Autodesk Fusion 360 part; units mm, degrees
(part 2 of 2)
  spline S357 degree 3 poles (-3.8049, -47.8973) (-3.3486, -49.266) (-3.3114, -49.4383) (-3.4138, -49.7828) knots 0 0 0 0 1 1 1 1
  spline S358 degree 3 poles (-3.4138, -49.7828) (-3.5255, -50.1506) (-3.4464, -50.4812) (-3.2508, -50.4812) knots 0 0 0 0 1 1 1 1
  spline S359 degree 3 poles (-3.2508, -50.4812) (-3.1484, -50.4812) (-3.1065, -50.416) (-3.0693, -50.2018) knots 0 0 0 0 1 1 1 1
  spline S360 degree 3 poles (-3.0693, -50.2018) (-3.032, -50.0249) (-3.0367, -50.0203) (-2.883, -50.5045) knots 0 0 0 0 1 1 1 1
  spline S361 degree 3 poles (-2.883, -50.5045) (-2.8225, -50.6814) (-2.7294, -50.9235) (-2.6689, -51.0399) knots 0 0 0 0 1 1 1 1
  spline S362 degree 3 poles (-2.6689, -51.0399) (-2.5385, -51.282) (-2.5292, -51.403) (-2.6316, -51.4449) knots 0 0 0 0 1 1 1 1
  spline S363 degree 3 poles (-2.6316, -51.4449) (-2.6735, -51.4589) (-2.9482, -51.4403) (-3.2415, -51.3984) knots 0 0 0 0 1 1 1 1
  spline S364 degree 3 poles (-3.2415, -51.3984) (-3.7863, -51.3192) (-4.303, -51.1237) (-4.4334, -50.9514) knots 0 0 0 0 1 1 1 1
  spline S365 degree 3 poles (-4.4334, -50.9514) (-4.466, -50.9095) (-4.587, -50.7978) (-4.7034, -50.7) knots 0 0 0 0 1 1 1 1
  spline S366 degree 3 poles (-4.7034, -50.7) (-4.9641, -50.4905) (-5.2156, -50.0249) (-5.2481, -49.6897) knots 0 0 0 0 1 1 1 1
  spline S367 degree 3 poles (-5.2481, -49.6897) (-5.29, -49.2474) (-4.9921, -48.158) (-4.7314, -47.8274) knots 0 0 0 0 1 1 1 1
  spline S368 degree 3 poles (-4.7314, -47.8274) (-4.466, -47.4783) (-4.1634, -47.1756) (-4.1028, -47.185) knots 0 0 0 0 1 1 1 1
  spline S369 degree 3 poles (-4.1028, -47.185) (-4.0656, -47.1943) (-3.9399, -47.5015) (-3.8049, -47.8973) knots 0 0 0 0 1 1 1 1
  spline S370 degree 3 poles (6.2235, -48.8005) (6.1909, -48.847) (5.9395, -48.9914) (5.2179, -49.3731) knots 0 0 0 0 1 1 1 1
  spline S371 degree 3 poles (5.2179, -49.3731) (4.9758, -49.5035) (4.7197, -49.6478) (4.6545, -49.6944) knots 0 0 0 0 1 1 1 1
  spline S372 degree 3 poles (4.6545, -49.6944) (4.5847, -49.7409) (4.5149, -49.7828) (4.5009, -49.7828) knots 0 0 0 0 1 1 1 1
  spline S373 degree 3 poles (4.5009, -49.7828) (4.4683, -49.7828) (4.026, -50.0482) (3.5185, -50.3695) knots 0 0 0 0 1 1 1 1
  spline S374 degree 3 poles (3.5185, -50.3695) (3.3416, -50.4812) (3.0902, -50.6348) (2.9645, -50.7047) knots 0 0 0 0 1 1 1 1
  spline S375 degree 3 poles (2.9645, -50.7047) (2.8388, -50.7745) (2.6619, -50.8955) (2.5688, -50.97) knots 0 0 0 0 1 1 1 1
  spline S376 degree 3 poles (2.5688, -50.97) (2.4757, -51.0492) (2.2569, -51.2028) (2.0753, -51.3146) knots 0 0 0 0 1 1 1 1
  spline S377 degree 3 poles (2.0753, -51.3146) (1.8984, -51.4263) (1.6982, -51.5567) (1.633, -51.6032) knots 0 0 0 0 1 1 1 1
  spline S378 degree 3 poles (1.633, -51.6032) (1.5678, -51.6498) (1.3909, -51.7662) (1.2373, -51.8639) knots 0 0 0 0 1 1 1 1
  spline S379 degree 3 poles (1.2373, -51.8639) (1.0836, -51.957) (0.916, -52.0781) (0.8648, -52.1247) knots 0 0 0 0 1 1 1 1
  spline S380 degree 3 poles (0.8648, -52.1247) (0.8136, -52.1712) (0.7158, -52.241) (0.6506, -52.2829) knots 0 0 0 0 1 1 1 1
  spline S381 degree 3 poles (0.6506, -52.2829) (0.3573, -52.4599) (0.3853, -52.6973) (0.6925, -52.6414) knots 0 0 0 0 1 1 1 1
  spline S382 degree 3 poles (0.6925, -52.6414) (0.8089, -52.6182) (0.8695, -52.6275) (0.9067, -52.674) knots 0 0 0 0 1 1 1 1
  spline S383 degree 3 poles (0.9067, -52.674) (1.0138, -52.809) (1.4468, -53.1396) (1.6051, -53.2048) knots 0 0 0 0 1 1 1 1
  spline S384 degree 3 poles (1.6051, -53.2048) (2.0054, -53.3724) (2.7224, -53.5074) (3.2206, -53.5074) knots 0 0 0 0 1 1 1 1
  spline S385 degree 3 poles (3.2206, -53.5074) (3.6955, -53.5074) (3.7187, -53.5027) (4.0819, -53.3258) knots 0 0 0 0 1 1 1 1
  spline S386 degree 3 poles (4.0819, -53.3258) (4.445, -53.1489) (4.6359, -53.0046) (4.9897, -52.6554) knots 0 0 0 0 1 1 1 1
  spline S387 degree 3 poles (4.9897, -52.6554) (5.162, -52.4878) (5.4972, -51.9803) (5.4972, -51.8919) knots 0 0 0 0 1 1 1 1
  spline S388 degree 3 poles (5.4972, -51.8919) (5.4972, -51.8686) (5.5577, -51.7243) (5.6322, -51.5706) knots 0 0 0 0 1 1 1 1
  spline S389 degree 3 poles (5.6322, -51.5706) (5.8138, -51.1935) (5.9255, -50.4626) (5.8836, -49.8666) knots 0 0 0 0 1 1 1 1
  line L38 (5.8836, -49.8666) -> (5.8557, -49.4243)
  line L39 (5.8557, -49.4243) -> (6.0187, -49.3033)
  spline S390 degree 3 poles (6.0187, -49.3033) (6.1071, -49.2335) (6.2002, -49.1776) (6.2282, -49.1776) knots 0 0 0 0 1 1 1 1
  spline S391 degree 3 poles (6.2282, -49.1776) (6.2514, -49.1776) (6.3213, -49.1264) (6.3818, -49.0612) knots 0 0 0 0 1 1 1 1
  spline S392 degree 3 poles (6.3818, -49.0612) (6.4703, -48.9634) (6.4842, -48.9215) (6.447, -48.861) knots 0 0 0 0 1 1 1 1
  spline S393 degree 3 poles (6.447, -48.861) (6.3865, -48.7679) (6.2608, -48.7353) (6.2235, -48.8005) knots 0 0 0 0 1 1 1 1
  spline S394 degree 3 poles (5.5298, -49.7177) (5.5438, -49.7596) (5.5345, -50.0668) (5.5019, -50.4067) knots 0 0 0 0 1 1 1 1
  spline S395 degree 3 poles (5.5019, -50.4067) (5.4507, -51.0352) (5.3203, -51.4915) (5.0596, -52.0036) knots 0 0 0 0 1 1 1 1
  spline S396 degree 3 poles (5.0596, -52.0036) (4.892, -52.3342) (4.4404, -52.7299) (3.9608, -52.972) knots 0 0 0 0 1 1 1 1
  spline S397 degree 3 poles (3.9608, -52.972) (3.742, -53.0837) (3.6303, -53.107) (3.2113, -53.1256) knots 0 0 0 0 1 1 1 1
  spline S398 degree 3 poles (3.2113, -53.1256) (2.8062, -53.1396) (2.6572, -53.1256) (2.3593, -53.0418) knots 0 0 0 0 1 1 1 1
  spline S399 degree 3 poles (2.3593, -53.0418) (1.7633, -52.8742) (1.1674, -52.5483) (1.1674, -52.3854) knots 0 0 0 0 1 1 1 1
  spline S400 degree 3 poles (1.1674, -52.3854) (1.1674, -52.3621) (1.2326, -52.3155) (1.3071, -52.2923) knots 0 0 0 0 1 1 1 1
  spline S401 degree 3 poles (1.3071, -52.2923) (1.3862, -52.2643) (1.4468, -52.2224) (1.4468, -52.1991) knots 0 0 0 0 1 1 1 1
  spline S402 degree 3 poles (1.4468, -52.1991) (1.4468, -52.1759) (1.5026, -52.1293) (1.5771, -52.1014) knots 0 0 0 0 1 1 1 1
  spline S403 degree 3 poles (1.5771, -52.1014) (1.647, -52.0688) (1.7633, -51.9943) (1.8332, -51.9384) knots 0 0 0 0 1 1 1 1
  spline S404 degree 3 poles (1.8332, -51.9384) (1.9077, -51.8779) (1.9868, -51.8313) (2.0101, -51.8313) knots 0 0 0 0 1 1 1 1
  spline S405 degree 3 poles (2.0101, -51.8313) (2.038, -51.8313) (2.1032, -51.7755) (2.1591, -51.7103) knots 0 0 0 0 1 1 1 1
  line L40 (2.1591, -51.7103) -> (2.2615, -51.5939)
  line L41 (2.2615, -51.5939) -> (2.2615, -51.8313)
  spline S406 degree 3 poles (2.2615, -51.8313) (2.2615, -52.0874) (2.3174, -52.1572) (2.4943, -52.12) knots 0 0 0 0 1 1 1 1
  spline S407 degree 3 poles (2.4943, -52.12) (2.62, -52.0967) (2.7131, -51.8919) (2.7829, -51.4822) knots 0 0 0 0 1 1 1 1
  spline S408 degree 3 poles (2.7829, -51.4822) (2.8202, -51.2401) (2.8295, -51.2308) (3.3137, -50.9468) knots 0 0 0 0 1 1 1 1
  spline S409 degree 3 poles (3.3137, -50.9468) (3.4254, -50.8816) (3.6908, -50.714) (3.9096, -50.5696) knots 0 0 0 0 1 1 1 1
  spline S410 degree 3 poles (3.9096, -50.5696) (4.1331, -50.4253) (4.4357, -50.2391) (4.5894, -50.1553) knots 0 0 0 0 1 1 1 1
  spline S411 degree 3 poles (4.5894, -50.1553) (4.743, -50.0715) (4.9059, -49.9737) (4.9525, -49.9318) knots 0 0 0 0 1 1 1 1
  spline S412 degree 3 poles (4.9525, -49.9318) (5.0736, -49.8247) (5.3669, -49.6525) (5.4414, -49.6478) knots 0 0 0 0 1 1 1 1
  spline S413 degree 3 poles (5.4414, -49.6478) (5.4739, -49.6432) (5.5112, -49.6758) (5.5298, -49.7177) knots 0 0 0 0 1 1 1 1
  spline S414 degree 3 poles (-7.2268, -49.6013) (-7.3246, -49.6571) (-7.3246, -49.7689) (-7.2315, -50.0948) knots 0 0 0 0 1 1 1 1
  spline S415 degree 3 poles (-7.2315, -50.0948) (-7.1616, -50.3369) (-7.1616, -50.3648) (-7.2548, -50.7093) knots 0 0 0 0 1 1 1 1
  spline S416 degree 3 poles (-7.2548, -50.7093) (-7.4084, -51.2773) (-7.3805, -52.3714) (-7.1896, -53.2048) knots 0 0 0 0 1 1 1 1
  spline S417 degree 3 poles (-7.1896, -53.2048) (-7.1384, -53.4189) (-6.9521, -53.8845) (-6.7659, -54.2523) knots 0 0 0 0 1 1 1 1
  spline S418 degree 3 poles (-6.7659, -54.2523) (-6.4074, -54.96) (-4.9409, -56.3613) (-4.2285, -56.6826) knots 0 0 0 0 1 1 1 1
  spline S419 degree 3 poles (-4.2285, -56.6826) (-4.1308, -56.7245) (-3.9958, -56.8036) (-3.9213, -56.8548) knots 0 0 0 0 1 1 1 1
  spline S420 degree 3 poles (-3.9213, -56.8548) (-3.7769, -56.9619) (-3.0739, -57.2459) (-2.3476, -57.4834) knots 0 0 0 0 1 1 1 1
  spline S421 degree 3 poles (-2.3476, -57.4834) (-1.5282, -57.7581) (-0.5878, -57.8977) (0.3992, -57.8931) knots 0 0 0 0 1 1 1 1
  spline S422 degree 3 poles (0.3992, -57.8931) (1.0091, -57.8931) (1.1721, -57.8744) (1.6702, -57.7534) knots 0 0 0 0 1 1 1 1
  spline S423 degree 3 poles (1.6702, -57.7534) (2.0753, -57.6556) (2.3174, -57.5672) (2.5083, -57.4554) knots 0 0 0 0 1 1 1 1
  spline S424 degree 3 poles (2.5083, -57.4554) (2.6526, -57.3623) (2.89, -57.232) (3.0297, -57.1621) knots 0 0 0 0 1 1 1 1
  spline S425 degree 3 poles (3.0297, -57.1621) (3.2951, -57.0271) (3.7001, -56.7291) (4.0074, -56.4405) knots 0 0 0 0 1 1 1 1
  spline S426 degree 3 poles (4.0074, -56.4405) (4.3147, -56.1518) (5.1713, -54.9739) (5.1713, -54.8389) knots 0 0 0 0 1 1 1 1
  spline S427 degree 3 poles (5.1713, -54.8389) (5.1713, -54.6853) (5.3063, -54.4944) (5.6881, -54.1033) knots 0 0 0 0 1 1 1 1
  spline S428 degree 3 poles (5.6881, -54.1033) (6.1164, -53.6703) (6.1956, -53.5353) (6.0559, -53.4608) knots 0 0 0 0 1 1 1 1
  spline S429 degree 3 poles (6.0559, -53.4608) (5.9907, -53.4236) (5.9162, -53.4655) (5.6788, -53.6797) knots 0 0 0 0 1 1 1 1
  spline S430 degree 3 poles (5.6788, -53.6797) (5.5158, -53.824) (5.3715, -53.9543) (5.3575, -53.973) knots 0 0 0 0 1 1 1 1
  spline S431 degree 3 poles (5.3575, -53.973) (5.2598, -54.1126) (4.054, -54.5596) (3.472, -54.676) knots 0 0 0 0 1 1 1 1
  spline S432 degree 3 poles (3.472, -54.676) (2.8062, -54.8063) (2.4012, -54.825) (1.6097, -54.7691) knots 0 0 0 0 1 1 1 1
  spline S433 degree 3 poles (1.6097, -54.7691) (0.4877, -54.6853) (-0.1781, -54.5922) (-0.6018, -54.4572) knots 0 0 0 0 1 1 1 1
  spline S434 degree 3 poles (-0.6018, -54.4572) (-0.8206, -54.392) (-1.1837, -54.2849) (-1.4118, -54.2244) knots 0 0 0 0 1 1 1 1
  spline S435 degree 3 poles (-1.4118, -54.2244) (-2.3989, -53.973) (-3.8747, -53.3398) (-4.3961, -52.9487) knots 0 0 0 0 1 1 1 1
  spline S436 degree 3 poles (-4.3961, -52.9487) (-4.5219, -52.8509) (-4.7127, -52.7252) (-4.8152, -52.6694) knots 0 0 0 0 1 1 1 1
  spline S437 degree 3 poles (-4.8152, -52.6694) (-5.0759, -52.525) (-5.2295, -52.3854) (-5.602, -51.9757) knots 0 0 0 0 1 1 1 1
  spline S438 degree 3 poles (-5.602, -51.9757) (-5.7789, -51.7801) (-6.0024, -51.5334) (-6.1001, -51.4263) knots 0 0 0 0 1 1 1 1
  spline S439 degree 3 poles (-6.1001, -51.4263) (-6.2026, -51.3192) (-6.2817, -51.2168) (-6.2817, -51.2028) knots 0 0 0 0 1 1 1 1
  spline S440 degree 3 poles (-6.2817, -51.2028) (-6.2817, -51.1842) (-6.3562, -51.0585) (-6.4493, -50.9188) knots 0 0 0 0 1 1 1 1
  spline S441 degree 3 poles (-6.4493, -50.9188) (-6.6542, -50.6115) (-6.9056, -50.1041) (-6.9847, -49.8387) knots 0 0 0 0 1 1 1 1
  spline S442 degree 3 poles (-6.9847, -49.8387) (-7.0546, -49.6013) (-7.1151, -49.5407) (-7.2268, -49.6013) knots 0 0 0 0 1 1 1 1
  spline S443 degree 3 poles (-6.7659, -51.2028) (-6.6681, -51.403) (-5.9791, -52.2085) (-5.8161, -52.3109) knots 0 0 0 0 1 1 1 1
  spline S444 degree 3 poles (-5.8161, -52.3109) (-5.6253, -52.4319) (-5.6206, -52.4086) (-5.9372, -53.3957) knots 0 0 0 0 1 1 1 1
  spline S445 degree 3 poles (-5.9372, -53.3957) (-5.9884, -53.5586) (-6.0536, -53.8566) (-6.156, -54.4153) knots 0 0 0 0 1 1 1 1
  spline S446 degree 3 poles (-6.156, -54.4153) (-6.17, -54.5037) (-6.2165, -54.4199) (-6.6635, -53.4701) knots 0 0 0 0 1 1 1 1
  spline S447 degree 3 poles (-6.6635, -53.4701) (-6.7938, -53.1955) (-6.9335, -52.3435) (-6.9661, -51.6172) knots 0 0 0 0 1 1 1 1
  spline S448 degree 3 poles (-6.9661, -51.6172) (-6.994, -50.97) (-6.9614, -50.7279) (-6.8776, -50.9468) knots 0 0 0 0 1 1 1 1
  spline S449 degree 3 poles (-6.8776, -50.9468) (-6.8544, -51.0119) (-6.8031, -51.1237) (-6.7659, -51.2028) knots 0 0 0 0 1 1 1 1
  spline S450 degree 3 poles (-5.2481, -52.7997) (-5.2388, -52.823) (-5.1038, -52.9254) (-4.9455, -53.0325) knots 0 0 0 0 1 1 1 1
  spline S451 degree 3 poles (-4.9455, -53.0325) (-4.7872, -53.1396) (-4.6476, -53.2467) (-4.6289, -53.2746) knots 0 0 0 0 1 1 1 1
  spline S452 degree 3 poles (-4.6289, -53.2746) (-4.587, -53.3444) (-4.0982, -53.6191) (-3.8561, -53.7076) knots 0 0 0 0 1 1 1 1
  spline S453 degree 3 poles (-3.8561, -53.7076) (-3.5255, -53.8333) (-3.4743, -53.9124) (-3.5348, -54.1871) knots 0 0 0 0 1 1 1 1
  spline S454 degree 3 poles (-3.5348, -54.1871) (-3.5628, -54.3128) (-3.6047, -54.4478) (-3.6233, -54.4851) knots 0 0 0 0 1 1 1 1
  spline S455 degree 3 poles (-3.6233, -54.4851) (-3.7071, -54.6434) (-3.9445, -55.6025) (-4.0237, -56.0773) knots 0 0 0 0 1 1 1 1
  spline S456 degree 3 poles (-4.0237, -56.0773) (-4.0563, -56.3008) (-4.1122, -56.3288) (-4.2704, -56.2077) knots 0 0 0 0 1 1 1 1
  spline S457 degree 3 poles (-4.2704, -56.2077) (-4.8105, -55.798) (-5.0247, -55.6257) (-5.1876, -55.4861) knots 0 0 0 0 1 1 1 1
  spline S458 degree 3 poles (-5.1876, -55.4861) (-5.29, -55.3976) (-5.3878, -55.3231) (-5.4064, -55.3231) knots 0 0 0 0 1 1 1 1
  spline S459 degree 3 poles (-5.4064, -55.3231) (-5.4204, -55.3231) (-5.5228, -55.216) (-5.6253, -55.0857) knots 0 0 0 0 1 1 1 1
  spline S460 degree 3 poles (-5.6253, -55.0857) (-5.7882, -54.8808) (-5.8161, -54.811) (-5.8161, -54.6294) knots 0 0 0 0 1 1 1 1
  spline S461 degree 3 poles (-5.8161, -54.6294) (-5.8161, -54.4013) (-5.7603, -54.1499) (-5.6532, -53.8799) knots 0 0 0 0 1 1 1 1
  spline S462 degree 3 poles (-5.6532, -53.8799) (-5.6206, -53.7914) (-5.5321, -53.5027) (-5.467, -53.2374) knots 0 0 0 0 1 1 1 1
  spline S463 degree 3 poles (-5.467, -53.2374) (-5.3506, -52.809) (-5.2947, -52.6926) (-5.2481, -52.7997) knots 0 0 0 0 1 1 1 1
  spline S464 degree 3 poles (-2.8784, -54.1313) (-2.5944, -54.2802) (-0.923, -54.7831) (-0.3597, -54.8901) knots 0 0 0 0 1 1 1 1
  spline S465 degree 3 poles (-0.3597, -54.8901) (0.0081, -54.96) (0.0454, -54.9786) (0.0268, -55.0671) knots 0 0 0 0 1 1 1 1
  spline S466 degree 3 poles (0.0268, -55.0671) (0.0175, -55.1183) (-0.0151, -55.3185) (-0.0431, -55.5093) knots 0 0 0 0 1 1 1 1
  spline S467 degree 3 poles (-0.0431, -55.5093) (-0.071, -55.7002) (-0.1455, -56.0448) (-0.206, -56.2775) knots 0 0 0 0 1 1 1 1
  spline S468 degree 3 poles (-0.206, -56.2775) (-0.2665, -56.5057) (-0.341, -56.8455) (-0.369, -57.0318) knots 0 0 0 0 1 1 1 1
  spline S469 degree 3 poles (-0.369, -57.0318) (-0.3969, -57.2133) (-0.4481, -57.3996) (-0.4854, -57.4461) knots 0 0 0 0 1 1 1 1
  spline S470 degree 3 poles (-0.4854, -57.4461) (-0.5412, -57.5253) (-0.5598, -57.5253) (-0.909, -57.4322) knots 0 0 0 0 1 1 1 1
  spline S471 degree 3 poles (-0.909, -57.4322) (-1.1139, -57.3763) (-1.3699, -57.3204) (-1.4863, -57.3018) knots 0 0 0 0 1 1 1 1
  spline S472 degree 3 poles (-1.4863, -57.3018) (-1.9472, -57.232) (-3.5907, -56.6733) (-3.735, -56.5383) knots 0 0 0 0 1 1 1 1
  spline S473 degree 3 poles (-3.735, -56.5383) (-3.7723, -56.501) (-3.5162, -55.393) (-3.2974, -54.6527) knots 0 0 0 0 1 1 1 1
  spline S474 degree 3 poles (-3.2974, -54.6527) (-3.2229, -54.4013) (-3.1624, -54.1638) (-3.1624, -54.1313) knots 0 0 0 0 1 1 1 1
  spline S475 degree 3 poles (-3.1624, -54.1313) (-3.1624, -54.0475) (-3.032, -54.0475) (-2.8784, -54.1313) knots 0 0 0 0 1 1 1 1
  spline S476 degree 3 poles (4.8128, -54.7598) (4.7244, -54.9088) (4.1471, -55.6723) (3.8491, -56.0494) knots 0 0 0 0 1 1 1 1
  spline S477 degree 3 poles (3.8491, -56.0494) (3.7839, -56.1286) (3.6117, -56.2868) (3.4627, -56.3939) knots 0 0 0 0 1 1 1 1
  spline S478 degree 3 poles (3.4627, -56.3939) (3.3137, -56.5057) (3.1228, -56.6593) (3.0437, -56.7385) knots 0 0 0 0 1 1 1 1
  spline S479 degree 3 poles (3.0437, -56.7385) (2.9599, -56.8129) (2.89, -56.8595) (2.89, -56.8316) knots 0 0 0 0 1 1 1 1
  spline S480 degree 3 poles (2.89, -56.8316) (2.89, -56.8083) (2.9505, -56.5429) (3.025, -56.2403) knots 0 0 0 0 1 1 1 1
  spline S481 degree 3 poles (3.025, -56.2403) (3.1042, -55.9377) (3.1787, -55.5745) (3.1973, -55.4349) knots 0 0 0 0 1 1 1 1
  spline S482 degree 3 poles (3.1973, -55.4349) (3.2113, -55.2952) (3.2392, -55.1741) (3.2578, -55.1602) knots 0 0 0 0 1 1 1 1
  spline S483 degree 3 poles (3.2578, -55.1602) (3.2764, -55.1509) (3.4999, -55.0996) (3.756, -55.0484) knots 0 0 0 0 1 1 1 1
  spline S484 degree 3 poles (3.756, -55.0484) (4.0493, -54.9879) (4.3286, -54.8948) (4.5195, -54.7924) knots 0 0 0 0 1 1 1 1
  spline S485 degree 3 poles (4.5195, -54.7924) (4.8966, -54.5968) (4.9199, -54.5922) (4.8128, -54.7598) knots 0 0 0 0 1 1 1 1
  spline S486 degree 3 poles (1.7959, -55.1648) (2.1265, -55.1788) (2.4384, -55.1741) (2.5641, -55.1415) knots 0 0 0 0 1 1 1 1
  spline S487 degree 3 poles (2.5641, -55.1415) (2.6805, -55.1183) (2.7876, -55.109) (2.8062, -55.1276) knots 0 0 0 0 1 1 1 1
  spline S488 degree 3 poles (2.8062, -55.1276) (2.8621, -55.1881) (2.6666, -56.1798) (2.485, -56.7804) knots 0 0 0 0 1 1 1 1
  spline S489 degree 3 poles (2.485, -56.7804) (2.4291, -56.9666) (2.3732, -57.0318) (2.2056, -57.1435) knots 0 0 0 0 1 1 1 1
  spline S490 degree 3 poles (2.2056, -57.1435) (2.0892, -57.2133) (1.8984, -57.2878) (1.7773, -57.3018) knots 0 0 0 0 1 1 1 1
  spline S491 degree 3 poles (1.7773, -57.3018) (1.6609, -57.3204) (1.4468, -57.367) (1.3071, -57.4042) knots 0 0 0 0 1 1 1 1
  spline S492 degree 3 poles (1.3071, -57.4042) (1.1674, -57.4461) (0.8043, -57.488) (0.497, -57.502) knots 0 0 0 0 1 1 1 1
  line L42 (0.497, -57.502) -> (-0.0524, -57.5253)
  line L43 (-0.0524, -57.5253) -> (-0.0291, -57.2971)
  spline S493 degree 3 poles (-0.0291, -57.2971) (-0.0058, -57.0411) (0.1106, -56.5289) (0.1897, -56.3288) knots 0 0 0 0 1 1 1 1
  spline S494 degree 3 poles (0.1897, -56.3288) (0.213, -56.2589) (0.2689, -55.9935) (0.3061, -55.7468) knots 0 0 0 0 1 1 1 1
  spline S495 degree 3 poles (0.3061, -55.7468) (0.4225, -55.0019) (0.362, -55.0764) (0.8322, -55.109) knots 0 0 0 0 1 1 1 1
  spline S496 degree 3 poles (0.8322, -55.109) (1.0557, -55.1229) (1.4887, -55.1509) (1.7959, -55.1648) knots 0 0 0 0 1 1 1 1
  spline S497 degree 3 poles (3.8072, -63.9269) (3.3742, -64.3226) (3.3649, -64.3272) (3.2858, -64.2621) knots 0 0 0 0 1 1 1 1
  spline S498 degree 3 poles (3.2858, -64.2621) (3.2485, -64.2295) (3.2159, -64.1596) (3.2159, -64.1038) knots 0 0 0 0 1 1 1 1
  spline S499 degree 3 poles (3.2159, -64.1038) (3.2113, -63.9641) (3.0763, -63.8058) (2.9226, -63.7686) knots 0 0 0 0 1 1 1 1
  spline S500 degree 3 poles (2.9226, -63.7686) (2.5874, -63.6894) (1.8518, -64.858) (1.8565, -65.4632) knots 0 0 0 0 1 1 1 1
  spline S501 degree 3 poles (1.8565, -65.4632) (1.8565, -65.6541) (1.8797, -65.7426) (1.9496, -65.8124) knots 0 0 0 0 1 1 1 1
  spline S502 degree 3 poles (1.9496, -65.8124) (2.0753, -65.9381) (2.1265, -65.8869) (2.1637, -65.6029) knots 0 0 0 0 1 1 1 1
  spline S503 degree 3 poles (2.1637, -65.6029) (2.2149, -65.2165) (2.3779, -64.7789) (2.5781, -64.4576) knots 0 0 0 0 1 1 1 1
  spline S504 degree 3 poles (2.5781, -64.4576) (2.6805, -64.2993) (2.7829, -64.169) (2.8062, -64.169) knots 0 0 0 0 1 1 1 1
  spline S505 degree 3 poles (2.8062, -64.169) (2.8248, -64.169) (2.8807, -64.2481) (2.9273, -64.3412) knots 0 0 0 0 1 1 1 1
  spline S506 degree 3 poles (2.9273, -64.3412) (2.9692, -64.439) (3.0204, -64.5274) (3.0344, -64.5414) knots 0 0 0 0 1 1 1 1
  spline S507 degree 3 poles (3.0344, -64.5414) (3.0483, -64.5554) (3.0856, -64.6112) (3.1182, -64.6671) knots 0 0 0 0 1 1 1 1
  spline S508 degree 3 poles (3.1182, -64.6671) (3.1461, -64.7276) (3.2066, -64.7742) (3.2532, -64.7742) knots 0 0 0 0 1 1 1 1
  spline S509 degree 3 poles (3.2532, -64.7742) (3.2951, -64.7742) (3.4999, -64.6159) (3.7001, -64.425) knots 0 0 0 0 1 1 1 1
  spline S510 degree 3 poles (3.7001, -64.425) (3.905, -64.2388) (4.0865, -64.0898) (4.1052, -64.1038) knots 0 0 0 0 1 1 1 1
  spline S511 degree 3 poles (4.1052, -64.1038) (4.1238, -64.1131) (4.1564, -64.2434) (4.1703, -64.3924) knots 0 0 0 0 1 1 1 1
  spline S512 degree 3 poles (4.1703, -64.3924) (4.2216, -64.8254) (4.2774, -64.9604) (4.4078, -64.9604) knots 0 0 0 0 1 1 1 1
  spline S513 degree 3 poles (4.4078, -64.9604) (4.5428, -64.9604) (4.6871, -64.8952) (4.8268, -64.7649) knots 0 0 0 0 1 1 1 1
  spline S514 degree 3 poles (4.8268, -64.7649) (4.9711, -64.6392) (4.9944, -64.7183) (4.8873, -64.9558) knots 0 0 0 0 1 1 1 1
  spline S515 degree 3 poles (4.8873, -64.9558) (4.7942, -65.1653) (4.7709, -65.3562) (4.8361, -65.3981) knots 0 0 0 0 1 1 1 1
  spline S516 degree 3 poles (4.8361, -65.3981) (4.8594, -65.412) (4.9385, -65.3841) (5.013, -65.3375) knots 0 0 0 0 1 1 1 1
  spline S517 degree 3 poles (5.013, -65.3375) (5.1899, -65.2305) (5.3808, -64.7509) (5.3343, -64.5368) knots 0 0 0 0 1 1 1 1
  spline S518 degree 3 poles (5.3343, -64.5368) (5.2831, -64.3133) (5.1713, -64.29) (4.8315, -64.425) knots 0 0 0 0 1 1 1 1
  spline S519 degree 3 poles (4.8315, -64.425) (4.6685, -64.4902) (4.5195, -64.5414) (4.5056, -64.5414) knots 0 0 0 0 1 1 1 1
  spline S520 degree 3 poles (4.5056, -64.5414) (4.4869, -64.5414) (4.473, -64.4157) (4.473, -64.2574) knots 0 0 0 0 1 1 1 1
  spline S521 degree 3 poles (4.473, -64.2574) (4.473, -64.006) (4.459, -63.9594) (4.3379, -63.8384) knots 0 0 0 0 1 1 1 1
  spline S522 degree 3 poles (4.3379, -63.8384) (4.2635, -63.7639) (4.1657, -63.7034) (4.1238, -63.7034) knots 0 0 0 0 1 1 1 1
  spline S523 degree 3 poles (4.1238, -63.7034) (4.0819, -63.7034) (3.9376, -63.8012) (3.8072, -63.9269) knots 0 0 0 0 1 1 1 1
extrude "Extrude29" cut sketch "Sketch8" against normal blind 31 contours A0 S107 S108 S109 S110 S111 S112 S113 S114 | A0 S78 S79 S80 S81 S82 S83 S84 S85 S86 S87 S88 S89 S90 | A0 S125 S126 S127 S128 | A0 S131 S132 L14 L15 S133 S134 S135 | A0 S67 S68 S69 S70 | A0 S139 S140 S141 S142 S143 S144 S145 S146 S147 S148 | A0 S149 S150 S151 S152 S153 S154 | A0 S55 S56 S57 S58 S59 S60 S61 S62 S63 S64 | A0 S4 L0 L1 S5 S6 S7 | A0 S28 S29 S30 S31 S32 S33 S34 S35 S36 S37 S38 S39 S40 S41
extrude "Extrude30" add sketch "Sketch8" against normal blind 14 contours A0 S211 S212 S213 S214 S215 S216 S217 S218 L20 L21 S219 L22 L23 S220 S221 S222 | A0 S90 S91 S92 S93 S94 S95 S96 S97 L10 L11 S98 S99 S100 S101 S102 S103 S104 S105 S106 S107 S211 S212 S213 S214 S215 S216 S217 S218 L20 L21 S219 L22 L23 S220 S221 S222 | A0 S114 S115 S116 S117 S118 S119 S120 S121 S122 S123 S124 L12 L13 S125 S188 S189 S190 S191 S192 S193 S194 S195 S196 S197 S198 | A0 S70 S71 S72 S73 S74 S75 S76 S77 S78 S239 S240 S241 S242 S243 S244 S245 S246 S247 S248 S249 | A0 S188 S189 S190 S191 S192 S193 S194 S195 S196 S197 S198 | A0 S239 S240 S241 S242 S243 S244 S245 S246 S247 S248 S249 S500 S501 S502 S503 S504 S505 S506 S507 S508 S509 S510 S511 S512 S513 S514 S515 S516 S517 S518 S519 S520 S521 S522 | A0 S497 S498 S499 S505 S506 S507 S508 S509 S510 S511 S512 S513 S514 S515 S516 S517 S518 S519 S520 S521 S522 S523 | A0 S497 S498 S499 S523 | A0 S128 S129 S130 S131 | A0 S135 S136 S137 S138 S139 S177 S178 S179 S180 | A0 S500 S501 S502 S503 S504 | A0 S177 S178 S179 S180 | A0 S64 S65 S66 S67 S339 S340 | A0 S339 S340 | A0 S0 S1 S2 S3 S4 S154 S155 S156 S157 S158 S159 S160 S161 S162 S163 S164 S330 S331 S332 S333 S334 | A0 S160 S161 S162 S163 S164 S330 S331 S332 S333 S334 | A0 S41 L6 L7 S42 S43 S44 S45 S46 S47 S48 S49 L8 L9 S50 S51 S52 S53 S54 S55 S271 S272 S273 S274 S275 S276 S277 S278 S279 S280 S281 | A0 S266 S267 S271 S272 S273 S274 S275 S276 S277 S278 S279 S280 S281 | A0 S266 S267 | A0 S7 S8 S9 S10 S11 S12 S13 S14 S15 S16 S17 S18 S19 S20 L2 L3 L4 L5 S21 S22 S23 S24 S25 S26 S27 S28 S302 S303 S304 S305 S306 S307 S308 L30 L31 S309 S310 S311 L32 L33 S312 S313 S314 | A0 S302 S303 S304 S305 S306 S307 S308 L30 L31 S309 S310 S311 L32 L33 S312 S313 S314
extrude "Extrude32" cut sketch "Sketch8" against normal blind 1.5 contours A0 S107 S108 S109 S110 S111 S112 S113 S114 S198 S199 S200 S201 S202 S203 S204 S205 S206 S207 S208 S209 S210 S211 | A0 S90 S91 S92 S93 S94 S95 S96 S97 L10 L11 S98 S99 S100 S101 S102 S103 S104 S105 S106 S107 S211 S212 S213 S214 S215 S216 S217 S218 L20 L21 S219 L22 L23 S220 S221 S222 | A0 S78 S79 S80 S81 S82 S83 S84 S85 S86 S87 S88 S89 S90 S222 S223 S224 S225 S226 S227 S228 S229 S230 S231 S232 S233 S234 S235 S236 S237 S238 L24 L25 S239 | A0 S114 S115 S116 S117 S118 S119 S120 S121 S122 S123 S124 L12 L13 S125 S188 S189 S190 S191 S192 S193 S194 S195 S196 S197 S198 | A0 S70 S71 S72 S73 S74 S75 S76 S77 S78 S239 S240 S241 S242 S243 S244 S245 S246 S247 S248 S249 | A0 S125 S126 S127 S128 S131 S132 L14 L15 S133 S134 S135 S180 S181 S182 S183 S184 L18 L19 S185 S186 S187 S188 | A0 S497 S498 S499 S505 S506 S507 S508 S509 S510 S511 S512 S513 S514 S515 S516 S517 S518 S519 S520 S521 S522 S523 | A0 S128 S129 S130 S131 | A0 S499 S500 S504 S505 | A0 S135 S136 S137 S138 S139 S177 S178 S179 S180 | A0 S500 S501 S502 S503 S504 | A0 S55 S56 S57 S58 S59 S60 S61 S62 S63 S64 S67 S68 S69 S70 S249 S250 L26 L27 S251 S252 S253 S254 S255 S256 S257 S258 S259 S260 S261 S262 S263 S264 S265 S266 S267 S268 S269 S270 S271 S335 S336 S337 S338 S339 S340 S341 S342 | A0 S139 S140 S141 S142 S143 S144 S145 S146 S147 S148 S149 S150 S151 S152 S153 S154 S164 S165 S166 S167 S168 S169 L16 L17 S170 S171 S172 S173 S174 S175 S176 S177 | A0 S64 S65 S66 S67 S339 S340 | A0 S0 S1 S2 S3 S4 S154 S155 S156 S157 S158 S159 S160 S161 S162 S163 S164 S330 S331 S332 S333 S334 | A0 S41 L6 L7 S42 S43 S44 S45 S46 S47 S48 S49 L8 L9 S50 S51 S52 S53 S54 S55 S271 S272 S273 S274 S275 S276 S277 S278 S279 S280 S281 | A0 S4 L0 L1 S5 S6 S7 S314 S315 S316 S317 S318 S319 S320 S321 S322 S323 S324 S325 S326 S327 S328 L34 L35 S329 S330 | A0 S266 S267 | A0 S7 S8 S9 S10 S11 S12 S13 S14 S15 S16 S17 S18 S19 S20 L2 L3 L4 L5 S21 S22 S23 S24 S25 S26 S27 S28 S302 S303 S304 S305 S306 S307 S308 L30 L31 S309 S310 S311 L32 L33 S312 S313 S314 | A0 S28 S29 S30 S31 S32 S33 S34 S35 S36 S37 S38 S39 S40 S41 S281 L28 L29 S282 S283 S284 S285 S286 S287 S288 S289 S290 S291 S292 S293 S294 S295 S296 S297 S298 S299 S300 S301 S302 | S343 L36 L37 S344 S345 S346 S347 S348 S349 S350 S351 S352 S353 S354 S355 S356 | S370 S371 S372 S373 S374 S375 S376 S377 S378 S379 S380 S381 S382 S383 S384 S385 S386 S387 S388 S389 L38 L39 S390 S391 S392 S393 | S414 S415 S416 S417 S418 S419 S420 S421 S422 S423 S424 S425 S426 S427 S428 S429 S430 S431 S432 S433 S434 S435 S436 S437 S438 S439 S440 S441 S442
